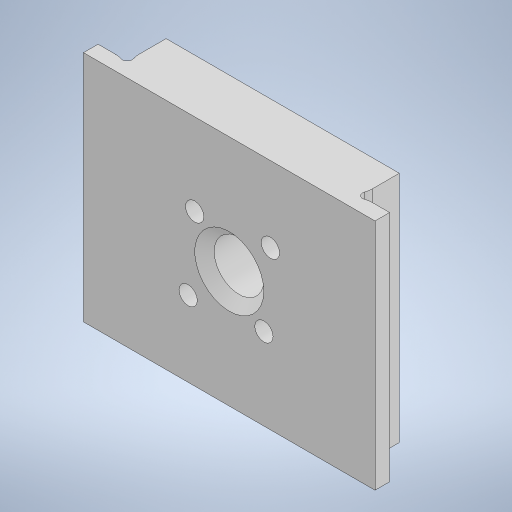
# Autodesk Inventor part: Drill Guide
Saved by Autodesk Inventor 2023.4 (Build 274418000, 418)
## iProperties
Created: 2024-05-04
Part Number: Drill Guide
Material: Generic
Document SubType Name: Modeling
Designer: Nathan Cai
Density: 1 g/cm^3
Appearance: Default
Author: Nathan Cai
Autodesk Inventor part; units mm, degrees
ref_plane "YZ Plane" through (0, 0, 0) normal (1, 0, 0) x (0, 1, 0)
ref_plane "XZ Plane" through (0, 0, 0) normal (0, 1, 0) x (-1, 0, 0)
ref_plane "XY Plane" through (0, 0, 0) normal (0, 0, 1) x (1, 0, 0)
sketch "Sketch1" plane through (0, 0, 0) normal (0, 0, 1) x (1, 0, 0)
  line L0 (-19.05, -19.05) -> (19.05, -19.05)
  line L1 (19.05, -19.05) -> (19.05, 19.05)
  line L2 (19.05, 19.05) -> (-19.05, 19.05)
  line L3 (-19.05, 19.05) -> (-19.05, -19.05)
  line L4 (-19.05, -19.05) -> (19.05, 19.05) construction
  line L5 (19.05, -19.05) -> (-19.05, 19.05) construction
  point P0 (0, 0)
  dimension "d0" = 38.1
  dimension "d1" = 38.1
  constraints: 12 end point, 2 midpoint, 2 parallel, 1 horizontal, 1 perpendicular
  measures "d0" distance of L2.end L1.end
  measures "d1" distance of L1.end L0.end
extrude "Extrusion1" add sketch "Sketch1" along normal blind 6.35
sketch "Sketch2" plane through (0, 0, 6.35) normal (0, 0, 1) x (1, 0, 0)
  line L0 (-23.8125, -19.05) -> (23.8125, -19.05)
  line L1 (23.8125, -19.05) -> (23.8125, 19.05)
  line L2 (23.8125, 19.05) -> (-23.8125, 19.05)
  line L3 (-23.8125, 19.05) -> (-23.8125, -19.05)
  line L4 (-23.8125, -19.05) -> (23.8125, 19.05) construction
  line L5 (23.8125, -19.05) -> (-23.8125, 19.05) construction
  point P0 (0, 0)
  point P1 (19.05, 19.05)
  dimension "d4" = 47.625
  constraints: 12 end point, 2 midpoint, 2 parallel, 1 horizontal, 1 perpendicular, 1 point on line
  measures "d4" distance of L2.end L1.end
extrude "Extrusion2" add sketch "Sketch2" along normal blind 2.3813
sketch "Sketch3" plane through (-19.05, 19.05, 0) normal (0, 1, 0) x (1, 0, 0)
  line L0 (0, 0) -> (0, -6.35) construction
  line L1 (0, -6.35) -> (-0.5613, -5.7887) construction
  line L2 (0, -6.35) -> (-4.7625, -6.35) construction
  circle A0 centre (-0.5613, -5.7887) radius 0.7937
  line L3 (19.05, 0) -> (19.05, -8.7313) construction
  line L4 (42.8625, -8.7313) -> (-4.7625, -8.7313) projected
  circle A1 centre (38.6613, -5.7887) radius 0.7937
  dimension "d8" = 1.5875
  dimension "d7" = 45
  constraints: 4 end point, 1 centre point, 1 coincident, 1 midpoint, 1 symmetric about line, 4 other
  measures "d7" angle of L0 L1
extrude "Extrusion3" cut sketch "Sketch3" against normal through all
fillet "Fillet1" radius 3.175 4 edges at (-19.05, 0, 5.2275) (-20.1725, 0, 6.35) (20.1725, 0, 6.35) (19.05, 0, 5.2275)
sketch "Sketch4" plane through (0, 0, 8.7313) normal (0, 0, 1) x (1, 0, 0)
  circle A0 centre (0, 0) radius 4.05
  circle A1 centre (0, 0) radius 8 construction
  circle A2 centre (0, 0) radius 9.5 construction
  line L0 (0, 0) -> (0, 9.5) construction
  line L1 (0, 0) -> (-5.6569, 5.6569) construction
  line L2 (0, 0) -> (-6.7175, -6.7175) construction
  circle A3 centre (-5.6569, 5.6569) radius 1.5
  circle A4 centre (-6.7175, -6.7175) radius 1.5
  circle A5 centre (6.7175, 6.7175) radius 1.5
  circle A6 centre (5.6569, -5.6569) radius 1.5
  dimension "d13" = 16
  dimension "d12" = 8.1
  dimension "d14" = 19
  dimension "d15" = 45
  dimension "d16" = 3
  dimension "d17" = 3
  dimension "d20" = 360
  constraints: 6 centre point, 6 end point, 5 coincident, 2 point on circle, 1 perpendicular, 1 vertical, 12 other
  measures "d12" diameter of A0
  measures "d14" diameter of A2
  measures "d15" angle of L0 L1
  measures "d16" diameter of A3
  measures "d17" diameter of A4
extrude "Extrusion4" cut sketch "Sketch4" against normal through all
chamfer "Chamfer1" distance 1.5875 angle 45 1 edges at (-4.05, 0, 8.7313)
body "Solid1"
